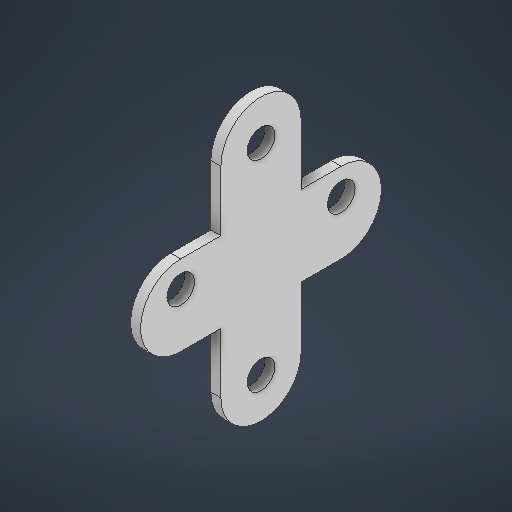
# Autodesk Inventor part: polygusset
Saved by Autodesk Inventor 2025.2 (Build 292293000, 293)
## iProperties
Created: 2025-04-08
Part Number: polygusset
Material: Generic
Document SubType Name: Modeling
Designer: roejo
Density: 1 g/cm^3
Appearance: Default
Author: roejo
Autodesk Inventor part; units mm, degrees
ref_plane "YZ Plane" through (0, 0, 0) normal (1, 0, 0) x (0, 1, 0)
ref_plane "XZ Plane" through (0, 0, 0) normal (0, 1, 0) x (-1, 0, 0)
ref_plane "XY Plane" through (0, 0, 0) normal (0, 0, 1) x (1, 0, 0)
sketch "Sketch1" plane through (0, 0, 0) normal (1, 0, 0) x (0, 1, 0)
  arc A0 (6.35, 0) -> (-6.35, 0) centre (0, 0) ccw
  arc A1 (-6.35, -25.4) -> (6.35, -25.4) centre (0, -25.4) ccw
  line L0 (-6.35, -19.05) -> (-15.875, -19.05)
  line L1 (-6.35, -6.35) -> (-15.875, -6.35)
  circle A2 centre (-15.875, -12.7) radius 2.1844
  arc A3 (-15.875, -6.35) -> (-15.875, -19.05) centre (-15.875, -12.7) ccw
  line L2 (-6.35, -25.4) -> (-6.35, -19.05)
  line L3 (-6.35, -6.35) -> (-6.35, 0)
  circle A4 centre (15.875, -12.7) radius 2.1844
  arc A5 (15.875, -19.05) -> (15.875, -6.35) centre (15.875, -12.7) ccw
  line L4 (15.875, -19.05) -> (6.35, -19.05)
  line L5 (15.875, -6.35) -> (6.35, -6.35)
  line L6 (6.35, 0) -> (6.35, -6.35)
  line L7 (6.35, -19.05) -> (6.35, -25.4)
  circle A6 centre (2.1844, 0) radius 2.1844
  circle A7 centre (2.1844, -25.4) radius 2.1844
  dimension "d18" = 6.35
  dimension "d20" = 4.3688
  dimension "d21" = 4.3688
  constraints: 16 end point, 8 centre point, 8 point on circle, 7 tangent, 4 perpendicular, 3 coincident, 2 horizontal
  measures "d18" distance of L3.end point (0, 0)
  measures "d20" diameter of A6
  measures "d21" diameter of A7
extrude "Extrusion1" add sketch "Sketch1" along normal blind 1.5875
body "Solid1"
